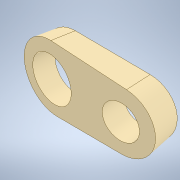
# Autodesk Inventor part: Крепление петли
Saved by Autodesk Inventor 2021.1 (Build 251245010, 245A)
## iProperties
Created: 2026-04-16
Part Number: Крепление петли
Material: Типовые
Document SubType Name: Modeling
Designer: Андрей Тарасов
Density: 1 g/cm^3
Appearance: По умолчанию
Author: Андрей Тарасов
Autodesk Inventor part; units mm, degrees
ref_plane "YZ Plane" through (0, 0, 0) normal (1, 0, 0) x (0, 1, 0)
ref_plane "XZ Plane" through (0, 0, 0) normal (0, 1, 0) x (-1, 0, 0)
ref_plane "XY Plane" through (0, 0, 0) normal (0, 0, 1) x (1, 0, 0)
sketch "Эскиз1" plane through (0, 0, 0) normal (0, 0, 1) x (1, 0, 0)
  circle A0 centre (0, 0) radius 6
  circle A1 centre (18, 0) radius 4
  line L0 (0, 0) -> (18, 0)
  line L1 (0, 0) -> (18, 0) construction
  line L2 (1, -8.9443) -> (18.7778, -6.9567)
  line L3 (18.7778, 6.9567) -> (1, 8.9443)
  arc A2 (1, 8.9443) -> (1, -8.9443) centre (0, 0) ccw
  arc A3 (18.7778, -6.9567) -> (18.7778, 6.9567) centre (18, 0) ccw
  point P0 (9, 0)
  dimension "d0" = 12
  dimension "d1" = 8
  dimension "d2" = 18
  dimension "d4" = 9
  dimension "d7" = 7
  constraints: 10 end point, 4 centre point, 4 point on circle, 4 tangent, 1 coincident, 1 collinear, 1 horizontal, 1 midpoint
  measures "d0" diameter of A0
  measures "d1" diameter of A1
  measures "d2" distance of L0.start L0.end
  measures "d4" radius of A2
  measures "d7" radius of A3
extrude "Выдавливание1" add sketch "Эскиз1" along normal blind 6
